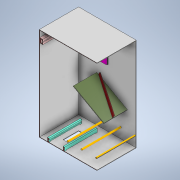
# Autodesk Inventor part: caja
Saved by Autodesk Inventor 2021.1 (Build 251245000, 245)
## iProperties
Created: 2020-12-31
Part Number: caja
Material: Generic
Document SubType Name: Modeling
Designer: Bolisteward
Density: 1 g/cm^3
Appearance: Default
Author: Bolisteward
Autodesk Inventor part; units mm, degrees
ref_plane "YZ Plane" through (0, 0, 0) normal (1, 0, 0) x (0, 1, 0)
ref_plane "XZ Plane" through (0, 0, 0) normal (0, 1, 0) x (-1, 0, 0)
ref_plane "XY Plane" through (0, 0, 0) normal (0, 0, 1) x (1, 0, 0)
sketch "Sketch1" plane through (0, 0, 0) normal (0, 0, 1) x (1, 0, 0)
  line L0 (0, 0) -> (400, 0)
  line L1 (400, 0) -> (400, 600)
  line L2 (400, 600) -> (0, 600)
  line L3 (0, 600) -> (0, 0)
  dimension "d0" = 400
  dimension "d1" = 600
  constraints: 8 end point, 2 parallel, 1 horizontal, 1 perpendicular
  measures "d0" distance of L2.end L1.end
  measures "d1" distance of L1.end L0.end
extrude "Extrusion1" add sketch "Sketch1" along normal blind 3
sketch "Sketch2" plane through (0, 0, 3) normal (0, 0, 1) x (1, 0, 0)
  line L0 (400, 600) -> (0, 600) projected
  line L1 (400, 0) -> (400, 600) projected
  line L2 (0, 600) -> (400, 600)
  line L3 (400, 600) -> (400, 0)
  line L4 (400, 0) -> (0, 0)
  line L5 (0, 0) -> (0, 600)
  line L6 (3, 597) -> (397, 597)
  line L7 (397, 597) -> (397, 3)
  line L8 (397, 3) -> (3, 3)
  line L9 (3, 3) -> (3, 597)
  dimension "d4" = 3
  constraints: 16 end point, 4 parallel, 2 perpendicular, 1 horizontal, 3 other
  measures "d4" distance between parallel lines of L5 L9
extrude "Extrusion2" add sketch "Sketch2" along normal blind 250
sketch "Sketch3" plane through (3, 597, 3) normal (0, -1, 0) x (1, 0, 0)
  line L0 (54, 110) -> (114, 110)
  line L1 (114, 110) -> (114, 70)
  line L2 (114, 70) -> (54, 70)
  line L3 (54, 70) -> (54, 110)
  line L4 (0, 250) -> (394, 250) projected
  line L5 (394, 0) -> (0, 0) projected
  point P0 (-3, -3)
  dimension "d7" = 40
  dimension "d8" = 60
  dimension "d9" = 54
  dimension "d11" = 70
  constraints: 8 end point, 2 parallel, 1 horizontal, 1 perpendicular
  measures "d7" distance of L0.end L1.end
  measures "d8" distance of L1.end L2.end
  measures "d9" distance from line of L3 L4.start
  measures "d11" distance between parallel lines of L5 L2
extrude "Extrusion3" add sketch "Sketch3" along normal blind 40
sketch "Sketch4" plane through (3, 557, 3) normal (0, -1, 0) x (1, 0, 0)
  circle A0 centre (104, 90) radius 5
  line L0 (114, 70) -> (114, 110) projected
  line L1 (114, 110) -> (54, 110) projected
  point P0 (-3, -3)
  dimension "d14" = 10
  dimension "d15" = 10
  dimension "d16" = 20
  constraints: 1 centre point
  measures "d14" diameter of A0
  measures "d15" distance from line of L0 A0.centre
  measures "d16" distance from line of A0.centre L1
extrude "Extrusion4" add sketch "Sketch4" along normal blind 30
sketch "Sketch5" plane through (0, 0, 253) normal (0, 0, 1) x (1, 0, 0)
  line L0 (3, 3) -> (3, 597) projected
  line L1 (3, 557) -> (23, 557)
  line L2 (23, 557) -> (23, 527)
  line L3 (23, 527) -> (3, 527)
  line L4 (3, 527) -> (3, 557)
  line L5 (23, 544.5) -> (18, 544.5)
  line L6 (18, 544.5) -> (18, 539.5)
  line L7 (18, 539.5) -> (23, 539.5)
  line L8 (23, 539.5) -> (23, 544.5)
  line L9 (23, 542) -> (-4.5465, 542) construction
  line L10 (18, 552) -> (13, 552)
  line L11 (13, 552) -> (13, 532)
  line L12 (13, 532) -> (18, 532)
  line L13 (18, 532) -> (18, 552)
  line L14 (3, 597) -> (397, 597) construction
  point P0 (0, 0)
  point P1 (18, 542)
  point P2 (18, 544.5)
  point P3 (3, 527)
  point P4 (23, 539.5)
  point P5 (18, 539.5)
  dimension "d19" = 20
  dimension "d20" = 30
  dimension "d21" = 5
  dimension "d22" = 5
  dimension "d24" = 2.5
  dimension "d25" = 5
  dimension "d26" = 20
  dimension "d28" = 10
  dimension "d29" = 40
  constraints: 26 end point, 6 parallel, 4 horizontal, 3 midpoint, 3 perpendicular, 2 point on line
  measures "d19" distance of L2.end L3.end
  measures "d20" distance of L1.end L2.end
  measures "d21" distance of L7.end L6.end
  measures "d22" distance of L6.end L5.end
  measures "d24" distance between parallel lines of L9 L5
  measures "d25" distance of L12.end L11.end
  measures "d26" distance of L11.end L10.end
  measures "d28" distance between parallel lines of L12 L9
  measures "d29" distance between parallel lines of L1 L14
extrude "Extrusion5" add sketch "Sketch5" against normal blind 250 contours L0 L1 L2 L5 L13 L10 L11 L12 L7 L3
sketch "Sketch6" plane through (0, 0, 3) normal (0, 0, 1) x (1, 0, 0)
  line L0 (148, 497) -> (193, 497)
  line L1 (193, 497) -> (193, 377)
  line L2 (193, 377) -> (148, 377)
  line L3 (148, 377) -> (148, 497)
  line L4 (3, 3) -> (3, 527) projected
  line L5 (3, 597) -> (397, 597) projected
  point P0 (0, 0)
  dimension "d32" = 45
  dimension "d33" = 120
  dimension "d34" = 145
  dimension "d35" = 100
  constraints: 8 end point, 2 parallel, 1 horizontal, 1 perpendicular
  measures "d32" distance of L1.end L2.end
  measures "d33" distance of L0.end L1.end
  measures "d34" distance between parallel lines of L4 L3
  measures "d35" distance between parallel lines of L5 L0
extrude "Extrusion6" add sketch "Sketch6" along normal blind 5
sketch "Sketch7" plane through (0, 0, 8) normal (0, 0, 1) x (1, 0, 0)
  line L0 (148, 377) -> (193, 377) projected
  line L1 (148, 497) -> (193, 497)
  line L2 (193, 497) -> (193, 377)
  line L3 (193, 377) -> (148, 377)
  line L4 (148, 377) -> (148, 497)
  line L5 (191, 495) -> (150, 495)
  line L6 (150, 495) -> (150, 379)
  line L7 (150, 379) -> (191, 379)
  line L8 (191, 379) -> (191, 495)
  point P0 (0, 0)
  point P1 (148, 377)
  dimension "d40" = 2
  constraints: 16 end point, 4 parallel, 2 perpendicular, 1 horizontal, 3 other
  measures "d40" distance between parallel lines of L1 L5
extrude "Extrusion7" add sketch "Sketch7" along normal blind 5 contours L8 L7 L6 L5
sketch "Sketch8" plane through (0, 0, 253) normal (0, 0, 1) x (1, 0, 0)
  line L0 (3, 527) -> (3, 3) projected
  line L1 (53, 26) -> (63, 26)
  line L2 (63, 26) -> (63, 6)
  line L3 (63, 6) -> (53, 6)
  line L4 (53, 6) -> (53, 26)
  line L5 (397, 3) -> (3, 3) projected
  line L6 (153, 26) -> (163, 26)
  line L7 (163, 26) -> (163, 6)
  line L8 (163, 6) -> (153, 6)
  line L9 (153, 6) -> (153, 26)
  line L10 (58, 16) -> (63, 16)
  line L11 (63, 16) -> (63, 11)
  line L12 (63, 11) -> (58, 11)
  line L13 (58, 11) -> (58, 16)
  line L14 (153, 16) -> (158, 16)
  line L15 (158, 16) -> (158, 11)
  line L16 (158, 11) -> (153, 11)
  line L17 (153, 11) -> (153, 16)
  point P0 (0, 0)
  point P1 (53, 28)
  dimension "d54" = 10
  dimension "d55" = 20
  dimension "d57" = 50
  dimension "d60" = 3
  dimension "d61" = 10
  dimension "d62" = 20
  dimension "d65" = 3
  dimension "d74" = 5
  dimension "d75" = 5
  dimension "d76" = 90
  dimension "d77" = 5
  dimension "d79" = 5
  dimension "d80" = 5
  dimension "d81" = 5
  constraints: 32 end point, 8 parallel, 4 horizontal, 4 perpendicular, 2 point on line, 1 midpoint
  measures "d54" distance of L2.end L3.end
  measures "d55" distance of L1.end L2.end
  measures "d57" distance between parallel lines of L4 L0
  measures "d60" distance between parallel lines of L5 L3
  measures "d61" distance of L7.end L8.end
  measures "d62" distance of L6.end L7.end
  measures "d65" distance between parallel lines of L5 L8
  measures "d74" distance of L10.end L11.end
  measures "d75" distance between parallel lines of L3 L12
  measures "d76" distance between parallel lines of L9 L2
  measures "d77" distance of L10.start L10.end
  measures "d79" distance of L15.end L16.end
  measures "d80" distance of L14.end L15.end
  measures "d81" distance between parallel lines of L8 L16
extrude "Extrusion8" add sketch "Sketch8" against normal blind 210 contours L1 L2 L10 L13 L12 L3 L4 | L6 L7 L8 L9 L16 L15 L14
sketch "Sketch9" plane through (53, 6, 253) normal (0, -1, 0) x (1, 0, 0)
  line L0 (0, 0) -> (0, -210) projected
  line L1 (10, 0) -> (10, -210) projected
  line L2 (0, 0) -> (10, 0)
  line L3 (10, 0) -> (10, -10)
  line L4 (10, -10) -> (0, -10)
  line L5 (0, -10) -> (0, 0)
  line L6 (100, 0) -> (110, 0) projected
  line L7 (110, 0) -> (110, -210) projected
  line L8 (100, 0) -> (110, 0)
  line L9 (110, 0) -> (110, -10)
  line L10 (110, -10) -> (100, -10)
  line L11 (100, -10) -> (100, 0)
  line L12 (10, -210) -> (0, -210) projected
  line L13 (0, -210) -> (10, -210)
  line L14 (10, -210) -> (10, -200)
  line L15 (10, -200) -> (0, -200)
  line L16 (0, -200) -> (0, -210)
  line L17 (110, -210) -> (100, -210) projected
  line L18 (100, -210) -> (110, -210)
  line L19 (110, -210) -> (110, -200)
  line L20 (110, -200) -> (100, -200)
  line L21 (100, -200) -> (100, -210)
  point P0 (-53, -253)
  point P1 (10, -200)
  point P2 (0, -200)
  dimension "d67" = 10
  dimension "d68" = 10
  dimension "d69" = 10
  dimension "d70" = 10
  dimension "d73" = 10
  constraints: 32 end point, 8 parallel, 4 horizontal, 4 perpendicular, 3 point on line
  measures "d67" distance of L2.end L3.end
  measures "d68" distance of L8.end L9.end
  measures "d69" distance of L14.end L13.end
  measures "d70" distance of L19.end L18.end
  measures "d73" distance between parallel lines of L19 L21
extrude "Extrusion9" add sketch "Sketch9" along normal blind 3 contours L2 L1 L4 L0 | L15 L1 L12 L0 | L7 L17 L21 L20 | L6 L7 L10 L11
sketch "Sketch10" plane through (3, 3, 3) normal (0, 1, 0) x (1, 0, 0)
  line L0 (90, -90) -> (120, -90)
  line L1 (120, -90) -> (120, -190)
  line L2 (120, -190) -> (90, -190)
  line L3 (90, -190) -> (90, -90)
  line L4 (50, -50) -> (60, -50) projected
  line L5 (60, -240) -> (50, -240) projected
  line L6 (60, -250) -> (60, -40) projected
  point P0 (-3, 3)
  dimension "d84" = 30
  dimension "d85" = 100
  dimension "d87" = 50
  dimension "d88" = 30
  constraints: 8 end point, 2 parallel, 1 horizontal, 1 perpendicular
  measures "d84" distance of L1.end L2.end
  measures "d85" distance of L0.end L1.end
  measures "d87" distance between parallel lines of L2 L5
  measures "d88" distance between parallel lines of L3 L6
extrude "Extrusion10" cut sketch "Sketch10" against normal blind 5
sketch "Sketch11" plane through (3, 3, 3) normal (0, 1, 0) x (1, 0, 0)
  line L0 (130, -130) -> (135, -130)
  line L1 (135, -130) -> (135, -150)
  line L2 (135, -150) -> (130, -150)
  line L3 (130, -150) -> (130, -130)
  line L4 (120, -90) -> (120, -190) projected
  line L5 (120, -190) -> (90, -190) projected
  point P0 (-3, 3)
  dimension "d91" = 5
  dimension "d92" = 20
  dimension "d93" = 10
  dimension "d94" = 40
  constraints: 8 end point, 2 parallel, 1 horizontal, 1 perpendicular
  measures "d91" distance of L1.end L2.end
  measures "d92" distance of L0.end L1.end
  measures "d93" distance between parallel lines of L3 L4
  measures "d94" distance between parallel lines of L2 L5
extrude "Extrusion11" add sketch "Sketch11" along normal blind 3
sketch "Sketch12" plane through (0, 0, 3) normal (0, 0, 1) x (1, 0, 0)
  line L0 (120.5173, 297) -> (317, 187.3663)
  line L1 (317, 187.3663) -> (314.5637, 183)
  line L2 (314.5637, 183) -> (118.081, 292.6337)
  line L3 (120.5173, 297) -> (118.081, 292.6337)
  line L4 (397, 597) -> (397, 3) projected
  line L5 (397, 3) -> (3, 3) projected
  line L6 (3, 597) -> (397, 597) projected
  point P0 (0, 0)
  point P1 (163, 3)
  dimension "d97" = 5
  dimension "d99" = 80
  dimension "d100" = 180
  dimension "d101" = 225
  dimension "d104" = 300
  constraints: 8 end point, 3 perpendicular
  measures "d97" distance of L0.end L1.end
  measures "d99" distance from line of L4 L0.end
  measures "d100" distance from line of L5 L1.end
  measures "d101" distance of L0.start L0.end
  measures "d104" distance from line of L0.start L6
extrude "Extrusion12" add sketch "Sketch12" along normal blind 150
sketch "Sketch13" plane through (3, 597, 3) normal (0, -1, 0) x (1, 0, 0)
  line L0 (174, 110) -> (214, 110)
  line L1 (214, 110) -> (214, 70)
  line L2 (214, 70) -> (174, 70)
  line L3 (174, 70) -> (174, 110)
  circle A0 centre (104, 90) radius 5 projected
  point P0 (-3, -3)
  dimension "d105" = 40
  dimension "d106" = 70
  constraints: 8 end point, 2 parallel, 1 horizontal, 1 perpendicular
  measures "d105" distance of L1.end L2.end
  measures "d106" distance from line of L3 A0.centre
extrude "Extrusion13" add sketch "Sketch13" along normal blind 40 contours L0 L1 L2 L3
sketch "Sketch15" plane through (3, 557, 3) normal (0, -1, 0) x (1, 0, 0)
  circle A0 centre (194, 90) radius 5
  circle A1 centre (194, 90) radius 2.5
  line L0 (174, 110) -> (174, 70) projected
  line L1 (214, 110) -> (174, 110) projected
  point P0 (-3, -3)
  dimension "d114" = 10
  dimension "d115" = 5
  dimension "d116" = 20
  dimension "d117" = 20
  constraints: 2 centre point, 1 coincident
  measures "d114" diameter of A0
  measures "d115" diameter of A1
  measures "d116" distance from line of A0.centre L0
  measures "d117" distance from line of L1 A0.centre
extrude "Extrusion15" add sketch "Sketch15" along normal blind 5
sketch "Sketch16" plane through (0, 0, 3) normal (0, 0, 1) x (1, 0, 0)
  circle A0 centre (183, 68) radius 5
  circle A1 centre (367, 68) radius 5
  line L0 (397, 597) -> (397, 3) projected
  line L1 (163, 3) -> (163, 26) projected
  line L2 (397, 3) -> (163, 3) projected
  circle A2 centre (273, 68) radius 5
  point P0 (0, 0)
  dimension "d120" = 10
  dimension "d121" = 10
  dimension "d122" = 30
  dimension "d123" = 20
  dimension "d124" = 65
  dimension "d125" = 65
  dimension "d128" = 10
  dimension "d129" = 90
  constraints: 3 centre point
  measures "d120" diameter of A0
  measures "d121" diameter of A1
  measures "d122" distance from line of L0 A1.centre
  measures "d123" distance from line of L1 A0.centre
  measures "d124" distance from line of L2 A0.centre
  measures "d125" distance from line of L2 A1.centre
  measures "d128" diameter of A2
  measures "d129" distance of A2.centre A0.centre
extrude "Extrusion16" add sketch "Sketch16" along normal blind 250
sketch "Sketch17" plane through (120.5173, 297, 153) normal (0.4873, 0.8733, 0) x (0.8733, -0.4873, 0)
  line L0 (225, 150) -> (225, 0) projected
  line L1 (225, 59.1442) -> (16.5288, 150)
  line L2 (-214.6928, 150) -> (40.632, 150) projected
  line L3 (11.5288, 150) -> (225, 54.1442)
  line L4 (225, 54.1442) -> (225, 59.1442)
  line L5 (11.5288, 150) -> (16.5288, 150)
  point P0 (39.474, 153)
  dimension "d132" = 5
  dimension "d133" = 5
  constraints: 8 end point, 3 point on line, 2 collinear
  measures "d132" distance of L1.start L3.end
  measures "d133" distance of L1.end L3.start
extrude "Extrusion17" add sketch "Sketch17" along normal blind 20
body "Solid1"
